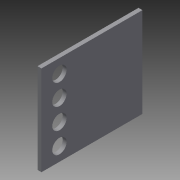
# Autodesk Inventor part: schreibtischplatte
Saved by Autodesk Inventor 2013 (Build 170138000, 138)
## iProperties
Created: 2014-03-29
Part Number: schreibtischplatte
Material: Generic
Document SubType Name: Modeling
Designer: hhanff
Density: 1 g/cm^3
Author: hhanff
Autodesk Inventor part; units mm, degrees
ref_plane "YZ Plane" through (0, 0, 0) normal (1, 0, 0) x (0, 1, 0)
ref_plane "XZ Plane" through (0, 0, 0) normal (0, 1, 0) x (-1, 0, 0)
ref_plane "XY Plane" through (0, 0, 0) normal (0, 0, 1) x (1, 0, 0)
sketch "Sketch4" plane through (0, 0, 0) normal (1, 0, 0) x (0, 1, 0)
  line L0 (0, 0) -> (562, 0)
  line L1 (562, 0) -> (562, 500)
  line L2 (562, 500) -> (0, 500)
  line L3 (0, 500) -> (0, 0)
  circle A0 centre (100, 424) radius 40
  circle A1 centre (100, 192) radius 40
  circle A2 centre (100, 76) radius 40
  circle A3 centre (100, 308) radius 40
  dimension "d31" = 562
  dimension "d33" = 500
  dimension "d34" = 80
  dimension "d35" = 80
  dimension "d36" = 80
  dimension "d37" = 80
  dimension "d39" = 100
  dimension "d40" = 100
  dimension "d41" = 100
  dimension "d42" = 100
  dimension "d50" = 76
  dimension "d51" = 192
  dimension "d52" = 76
  dimension "d53" = 192
  constraints: 8 end point, 4 centre point, 2 parallel, 1 horizontal, 1 perpendicular
  measures "d31" distance of L1.end L2.end
  measures "d33" distance of L2.end L0.start
  measures "d34" diameter of A0
  measures "d35" diameter of A1
  measures "d36" diameter of A2
  measures "d37" diameter of A3
  measures "d39" distance from line of L3 A0.centre
  measures "d40" distance from line of L3 A3.centre
  measures "d41" distance from line of L3 A1.centre
  measures "d42" distance from line of L3 A2.centre
  measures "d50" distance from line of L0 A2.centre
  measures "d51" distance from line of L0 A1.centre
  measures "d52" distance from line of L2 A0.centre
  measures "d53" distance from line of L2 A3.centre
extrude "Extrusion2" add sketch "Sketch4" along normal blind 22
body "Solid2"
